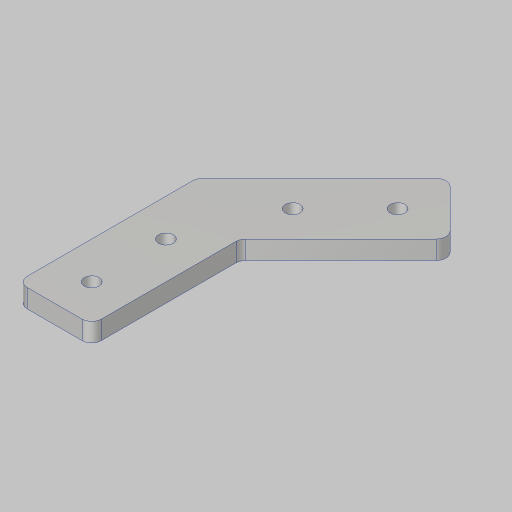
# Autodesk Inventor part: CL3-009
Saved by Autodesk Inventor 2023.5 (Build 275446000, 446)
## iProperties
Created: 2025-01-31
Part Number: CL3-009
Material: Aluminum 6061
Document SubType Name: Modeling
Designer: brand
Density: 2.7 g/cm^3
Appearance: Aluminum - Flat
Author: brand
Autodesk Inventor part; units mm, degrees
ref_plane "YZ Plane" through (0, 0, 0) normal (1, 0, 0) x (0, 1, 0)
ref_plane "XZ Plane" through (0, 0, 0) normal (0, 1, 0) x (-1, 0, 0)
ref_plane "XY Plane" through (0, 0, 0) normal (0, 0, 1) x (1, 0, 0)
sketch "Sketch1" plane through (0, 0, 0) normal (0, 1, 0) x (-1, 0, 0)
  line L0 (-12.7, 0) -> (12.7, 0)
  line L1 (12.7, 0) -> (12.7, -61.321)
  line L2 (12.7, -61.321) -> (-30.6605, -104.6815)
  line L3 (-30.6605, -104.6815) -> (-48.621, -86.721)
  line L4 (-48.621, -86.721) -> (-12.7, -50.8)
  line L5 (-12.7, -50.8) -> (-12.7, 0)
  point P0 (0, 0)
  point P1 (0, 0)
  dimension "d0" = 25.4
  dimension "d2" = 25.4
  dimension "d4" = 135
  dimension "d8" = 50.8
  dimension "d9" = 50.8
  constraints: 12 end point, 4 perpendicular, 1 coincident, 1 horizontal, 1 midpoint
  measures "d0" distance of L0.start L0.end
  measures "d2" distance of L2.end L3.end
  measures "d4" angle of L5 L4
  measures "d8" distance of L4.end L0.start
  measures "d9" distance of L3.end L4.end
extrude "Extrusion1" add sketch "Sketch1" along normal mid plane 6.35
sketch "Sketch2" plane through (0, 3.175, 0) normal (0, 1, 0) x (1, 0, 0)
  line L0 (12.7, 50.8) -> (12.7, 0) construction
  line L1 (12.7, 0) -> (-12.7, 0) construction
  line L2 (-12.7, 0) -> (-12.7, 61.321) construction
  line L3 (-12.7, 61.321) -> (30.6605, 104.6815) construction
  line L4 (30.6605, 104.6815) -> (48.621, 86.721) construction
  line L5 (48.621, 86.721) -> (12.7, 50.8) construction
  line L6 (48.621, 86.721) -> (30.6605, 104.6815) construction
  line L7 (39.6408, 95.7013) -> (0, 56.0605) construction
  line L8 (0, 56.0605) -> (0, 0) construction
  line L9 (-12.7, 0) -> (12.7, 0) construction
  point P0 (0, 0)
  point P1 (0, 12.7)
  point P2 (0, 38.1)
  point P3 (30.6605, 86.721)
  point P4 (12.7, 68.7605)
  dimension "d12" = 25.4
  dimension "d13" = 12.7
  dimension "d14" = 25.4
  dimension "d15" = 12.7
  constraints: 4 end point, 4 point on line, 3 midpoint, 2 perpendicular
  measures "d12" distance of point (0, 12.7) point (0, 38.1)
  measures "d13" distance from line of L1 point (0, 12.7)
  measures "d14" distance of point (30.661, 86.721) point (12.7, 68.761)
  measures "d15" distance from line of L4 point (30.661, 86.721)
hole "Hole1" at (0, 3.175, -12.7) at (0, 3.175, -38.1) at (30.6605, 3.175, -86.721) at (12.7, 3.175, -68.7605) direction (0, -1, 0) diameter 5.1054 end through all clearance for "Flat Head Machine Screw (82)" size "#10" standard "Ansi Unified Screw Threads"
fillet "Fillet1" radius 3.302 6 edges at (12.7, 0, -50.8) (-12.7, 0, -61.321) (48.621, 0, -86.721) (30.6605, 0, -104.6815) (12.7, 0, 0) (-12.7, 0, 0)
equation "\"d2\" = d0"
equation "\"d14\" = d12"
equation "\"d15\" = d13"
body "Solid1"
